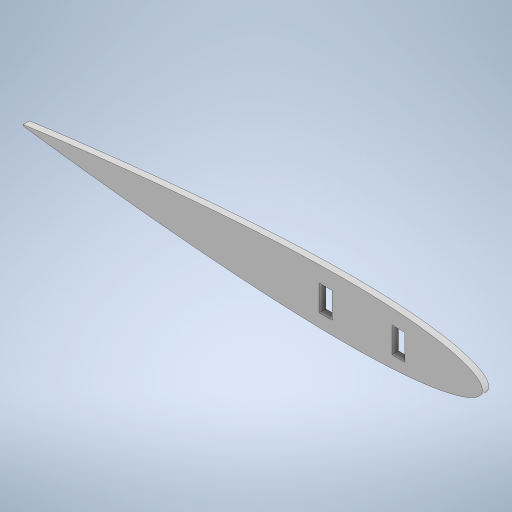
# Autodesk Inventor part: back side foil
Saved by Autodesk Inventor 2024 (Build 280153000, 153)
## iProperties
Created: 2023-07-07
Part Number: back side foil
Material: Generic
Document SubType Name: Modeling
Designer: USER
Density: 1 g/cm^3
Appearance: Default
Author: USER
Autodesk Inventor part; units mm, degrees
ref_plane "YZ Plane" through (0, 0, 0) normal (1, 0, 0) x (0, 1, 0)
ref_plane "XZ Plane" through (0, 0, 0) normal (0, 1, 0) x (-1, 0, 0)
ref_plane "XY Plane" through (0, 0, 0) normal (0, 0, 1) x (1, 0, 0)
sketch "Sketch1" plane through (0, 0, 0) normal (0, 0, 1) x (1, 0, 0)
  line L0 (64.6506, 7.1117) -> (59.6506, 7.1117)
  line L1 (59.6506, 7.1117) -> (59.6506, -2.8883)
  line L2 (64.6506, -2.8883) -> (64.6506, 7.1117)
  line L3 (59.6506, -2.8883) -> (64.6506, -2.8883)
  line L4 (36.1323, 5.6773) -> (31.1323, 5.6773)
  line L5 (36.1323, -4.3227) -> (36.1323, 5.6773)
  line L6 (31.1323, 5.6773) -> (31.1323, -4.3227)
  line L7 (31.1323, -4.3227) -> (36.1323, -4.3227)
  line L8 (-84.9715, 2.4164) -> (-84.9715, 2.87)
  spline S0 degree 4 poles (-84.9715, 2.87) (-84.9072, 2.879) (-84.5934, 2.923) (-84.067, 2.9966) (-83.1794, 3.12) (-82.2477, 3.2488) (-81.1059, 3.4055) (-79.765, 3.5881) (-78.2246, 3.7957) (-76.4903, 4.027) (-74.5651, 4.2805) (-72.4542, 4.555) (-70.1621, 4.8486) (-67.6945, 5.1599) (-65.057, 5.4872) (-62.2558, 5.8288) (-59.2974, 6.1828) (-56.1888, 6.5476) (-52.9372, 6.9214) (-49.5502, 7.3024) (-46.0357, 7.6887) (-42.402, 8.0786) (-38.6575, 8.4701) (-34.811, 8.8614) (-30.8714, 9.2505) (-26.848, 9.6354) (-22.7501, 10.0142) (-18.5873, 10.3848) (-14.3694, 10.7449) (-10.1062, 11.0925) (-5.8076, 11.4252) (-1.4838, 11.7408) (2.8553, 12.037) (7.1995, 12.3115) (11.5387, 12.5619) (15.8626, 12.7858) (20.1613, 12.9811) (24.4246, 13.1455) (28.6427, 13.2769) (32.8057, 13.3734) (36.9038, 13.4331) (40.9275, 13.4545) (44.8674, 13.4362) (48.7144, 13.377) (52.4594, 13.2761) (56.0936, 13.1329) (59.6087, 12.9471) (62.9964, 12.7186) (66.2488, 12.448) (69.3584, 12.1358) (72.3179, 11.7828) (75.1204, 11.3904) (77.7595, 10.96) (80.2291, 10.4932) (82.5234, 9.9918) (84.6374, 9.4579) (86.5664, 8.8935) (88.3062, 8.3006) (89.8534, 7.6812) (91.2051, 7.0371) (92.3595, 6.3694) (93.3153, 5.6781) (94.0712, 4.9618) (94.6232, 4.2168) (94.962, 3.4433) (95.0749, 2.6432) (94.962, 1.8431) (94.6232, 1.0695) (94.0712, 0.3245) (93.3153, -0.3917) (92.3595, -1.083) (91.2051, -1.7508) (89.8534, -2.3949) (88.3062, -3.0143) (86.5664, -3.6071) (84.6374, -4.1716) (82.5234, -4.7055) (80.2291, -5.2068) (77.7595, -5.6736) (75.1204, -6.1041) (72.3179, -6.4965) (69.3584, -6.8494) (66.2488, -7.1616) (62.9964, -7.4323) (59.6087, -7.6607) (56.0936, -7.8465) (52.4594, -7.9898) (48.7144, -8.0907) (44.8674, -8.1499) (40.9275, -8.1682) (36.9038, -8.1468) (32.8057, -8.087) (28.6427, -7.9905) (24.4246, -7.8591) (20.1613, -7.6947) (15.8626, -7.4995) (11.5387, -7.2755) (7.1995, -7.0251) (2.8553, -6.7507) (-1.4838, -6.4545) (-5.8076, -6.1388) (-10.1062, -5.8061) (-14.3694, -5.4586) (-18.5873, -5.0984) (-22.7501, -4.7279) (-26.848, -4.3491) (-30.8714, -3.9642) (-34.811, -3.5751) (-38.6575, -3.1838) (-42.402, -2.7922) (-46.0357, -2.4024) (-49.5502, -2.0161) (-52.9372, -1.6351) (-56.1888, -1.2613) (-59.2974, -0.8965) (-62.2558, -0.5424) (-65.057, -0.2008) (-67.6945, 0.1264) (-70.1621, 0.4377) (-72.4542, 0.7314) (-74.5651, 1.0058) (-76.4903, 1.2594) (-78.2246, 1.4906) (-79.765, 1.6983) (-81.1059, 1.8808) (-82.2477, 2.0375) (-83.1794, 2.1663) (-84.067, 2.2897) (-84.5934, 2.3634) (-84.9072, 2.4073) (-84.9715, 2.4164) knots -1 -1 -1 -1 -1 -0.9937 -0.989993 -0.98568 -0.980849 -0.975559 -0.969852 -0.963765 -0.957328 -0.950566 -0.943503 -0.936159 -0.928552 -0.920701 -0.912622 -0.90433 -0.895841 -0.887169 -0.878328 -0.869332 -0.860192 -0.850923 -0.841536 -0.832045 -0.822461 -0.812797 -0.803064 -0.793274 -0.78344 -0.773572 -0.763683 -0.753783 -0.743886 -0.734001 -0.724142 -0.714318 -0.704542 -0.694826 -0.68518 -0.675617 -0.666148 -0.656784 -0.647538 -0.638421 -0.629445 -0.620622 -0.611965 -0.603485 -0.595196 -0.587111 -0.579243 -0.571605 -0.564212 -0.557077 -0.550216 -0.543644 -0.537373 -0.531419 -0.52579 -0.520492 -0.515517 -0.510839 -0.506398 -0.502114 -0.497886 -0.493602 -0.489161 -0.484483 -0.479508 -0.47421 -0.468581 -0.462627 -0.456356 -0.449784 -0.442923 -0.435788 -0.428395 -0.420757 -0.412889 -0.404804 -0.396515 -0.388035 -0.379378 -0.370555 -0.361579 -0.352462 -0.343216 -0.333852 -0.324383 -0.31482 -0.305174 -0.295458 -0.285682 -0.275858 -0.265999 -0.256114 -0.246217 -0.236317 -0.226428 -0.21656 -0.206726 -0.196936 -0.187203 -0.177539 -0.167955 -0.158464 -0.149077 -0.139808 -0.130668 -0.121672 -0.112831 -0.104159 -0.09567 -0.087378 -0.079299 -0.071448 -0.063841 -0.056497 -0.049434 -0.042672 -0.036235 -0.030148 -0.024441 -0.019151 -0.01432 -0.010007 -0.0063 0 0 0 0 0
  point P0 (0, 0)
  constraints: 18 end point, 2 other
extrude "Extrusion1" add sketch "Sketch1" along normal blind 2.5
sketch "Sketch3" plane through (0, 0, 2.5) normal (0, 0, 1) x (1, 0, 0)
  line L0 (59.6506, 7.1117) -> (64.6506, 7.1117) projected
  line L1 (59.6506, 7.1117) -> (64.6506, 7.1117) projected
  line L2 (64.6506, 7.1117) -> (64.6506, -2.8883) projected
  line L3 (64.6506, 7.1117) -> (64.6506, -2.8883) projected
  line L4 (59.6506, -2.8883) -> (59.6506, 7.1117) projected
  line L5 (59.6506, -2.8883) -> (59.6506, 7.1117) projected
  line L6 (64.6506, -2.8883) -> (59.6506, -2.8883) projected
  line L7 (64.6506, -2.8883) -> (59.6506, -2.8883) projected
  line L8 (31.1323, 7.1117) -> (36.1323, 7.1117)
  line L9 (36.1323, 7.1117) -> (36.1323, -2.8883)
  line L10 (36.1323, -2.8883) -> (31.1323, -2.8883)
  line L11 (31.1323, -2.8883) -> (31.1323, 7.1117)
  point P0 (0, 0)
  constraints: 8 end point, 2 parallel, 1 horizontal, 1 perpendicular
extrude "Extrusion2" cut sketch "Sketch3" against normal blind 10 contours L8 L9 L10 L11
sketch "Sketch4" plane through (0, 0, 2.5) normal (0, 0, 1) x (1, 0, 0)
  line L0 (31.1323, -2.8883) -> (36.1323, -2.8883)
  line L1 (36.1323, -2.8883) -> (36.1323, -4.3227)
  line L2 (36.1323, -4.3227) -> (31.1323, -4.3227)
  line L3 (31.1323, -4.3227) -> (31.1323, -2.8883)
  point P0 (0, 0)
  constraints: 8 end point, 2 parallel, 1 horizontal, 1 perpendicular
extrude "Extrusion3" add sketch "Sketch4" against normal blind 2.5
body "Solid1"
